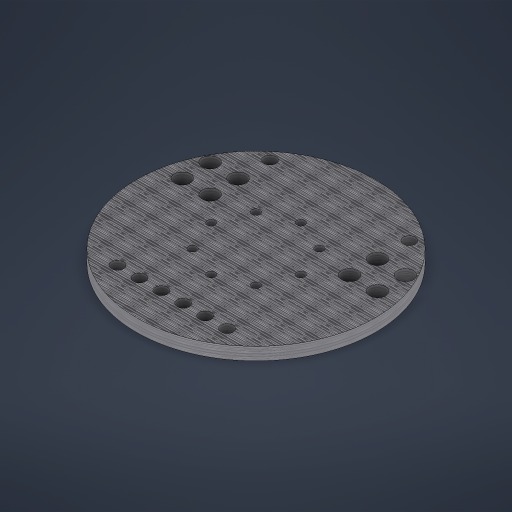
# Autodesk Inventor part: TurretBasePlate
Saved by Autodesk Inventor 2024 (Build 280153000, 153)
## iProperties
Created: 2023-11-22
Part Number: TurretBasePlate
Material: Generic
Document SubType Name: Modeling
Designer: avsar
Density: 1 g/cm^3
Appearance: Machined 03
Author: avsar
Autodesk Inventor part; units mm, degrees
ref_plane "YZ Plane" through (0, 0, 0) normal (1, 0, 0) x (0, 1, 0)
ref_plane "XZ Plane" through (0, 0, 0) normal (0, 1, 0) x (-1, 0, 0)
ref_plane "XY Plane" through (0, 0, 0) normal (0, 0, 1) x (1, 0, 0)
sketch "Sketch1" plane through (0, 0, 0) normal (0, 1, 0) x (-1, 0, 0)
  circle A0 centre (0, 0) radius 60
  dimension "d0" = 120
  constraints: 1 centre point, 1 coincident
  measures "d0" diameter of A0
extrude "Extrusion1" add sketch "Sketch1" along normal mid plane 6.35
sketch "Sketch2" plane through (0, 3.175, 0) normal (0, 1, 0) x (1, 0, 0)
  circle A0 centre (0, 22.5) radius 2
  circle A1 centre (-15.9099, 15.9099) radius 2
  circle A2 centre (-22.5, 0) radius 2
  circle A3 centre (-15.9099, -15.9099) radius 2
  circle A4 centre (0, -22.5) radius 2
  circle A5 centre (15.9099, -15.9099) radius 2
  circle A6 centre (22.5, 0) radius 2
  circle A7 centre (15.9099, 15.9099) radius 2
  point P0 (0, 0)
  dimension "d3" = 4
  dimension "d4" = 22.5
  dimension "d7" = 360
  constraints: 8 centre point, 1 vertical alignment, 17 other
  measures "d3" diameter of A0
  measures "d4" distance of point (0, 0) A0.centre
extrude "Extrusion2" cut sketch "Sketch2" against normal through all
sketch "Sketch3" plane through (0, 3.175, 0) normal (0, 1, 0) x (1, 0, 0)
  circle A0 centre (-42, 20) radius 2.5 construction
  circle A1 centre (-48, 26) radius 2 construction
  circle A2 centre (-48, 14) radius 2 construction
  circle A3 centre (-36, 14) radius 2 construction
  circle A4 centre (-36, 26) radius 2 construction
  circle A5 centre (0, 0) radius 60 construction
  line L0 (0, 60) -> (0, -60) construction
  circle A6 centre (42, 20) radius 2.5 construction
  circle A7 centre (48, 26) radius 2 construction
  circle A8 centre (48, 14) radius 2 construction
  circle A9 centre (36, 14) radius 2 construction
  circle A10 centre (36, 26) radius 2 construction
  circle A11 centre (-20, -42) radius 2.5 construction
  circle A12 centre (-25, -37) radius 2 construction
  circle A13 centre (-25, -47) radius 2 construction
  circle A14 centre (-15, -47) radius 2 construction
  circle A15 centre (-15, -37) radius 2 construction
  circle A16 centre (20, -42) radius 2.5 construction
  circle A17 centre (25, -37) radius 2 construction
  circle A18 centre (25, -47) radius 2 construction
  circle A19 centre (15, -47) radius 2 construction
  circle A20 centre (15, -37) radius 2 construction
  circle A21 centre (-27.5, -42) radius 3
  line L1 (-60, 0) -> (60, 0) construction
  circle A22 centre (-16.5, -42) radius 3
  circle A23 centre (-5.5, -42) radius 3
  circle A24 centre (5.5, -42) radius 3
  circle A25 centre (16.5, -42) radius 3
  circle A26 centre (27.5, -42) radius 3
  line L2 (-5.5, -42) -> (5.5, -42) construction
  point P0 (0, -42)
  dimension "d11" = 5
  dimension "d12" = 42
  dimension "d13" = 20
  dimension "d14" = 4
  dimension "d15" = 6
  dimension "d16" = 6
  dimension "d19" = 360
  dimension "d23" = 5
  dimension "d24" = 42
  dimension "d25" = 20
  dimension "d26" = 4
  dimension "d27" = 5
  dimension "d28" = 5
  dimension "d31" = 360
  dimension "d49" = 6
  dimension "d52" = 11
  constraints: 26 centre point, 10 symmetric about line, 6 end point, 4 point on circle, 3 horizontal, 3 midpoint, 1 coincident, 1 horizontal alignment, 1 vertical, 1 vertical alignment, 38 other
  measures "d11" diameter of A0
  measures "d12" horizontal distance of point (0, 0) A0.centre
  measures "d13" vertical distance of point (0, 0) A0.centre
  measures "d14" diameter of A1
  measures "d15" horizontal distance of A1.centre A0.centre
  measures "d16" horizontal distance of A0.centre A1.centre
  measures "d23" diameter of A11
  measures "d24" vertical distance of point (0, 0) A11.centre
  measures "d25" horizontal distance of point (0, 0) A11.centre
  measures "d26" diameter of A12
  measures "d27" horizontal distance of A11.centre A12.centre
  measures "d28" horizontal distance of A11.centre A12.centre
  measures "d49" diameter of A21
  measures "d52" distance of A21.centre A22.centre
extrude "Extrusion3" cut sketch "Sketch3" against normal through all
sketch "Sketch4" plane through (0, 3.175, 0) normal (0, 1, 0) x (1, 0, 0)
  circle A0 centre (-49, 42) radius 3 construction
  circle A1 centre (-49, 26) radius 4
  circle A2 centre (-49, 12) radius 4
  circle A3 centre (0, 0) radius 60 construction
  line L0 (-60, 0) -> (60, 0) construction
  circle A4 centre (-35, 42) radius 3
  circle A5 centre (-35, 26) radius 4
  circle A6 centre (-35, 12) radius 4
  line L1 (0, 60) -> (0, 0) construction
  circle A7 centre (49, 26) radius 4
  circle A8 centre (49, 12) radius 4
  circle A9 centre (35, 42) radius 3
  circle A10 centre (35, 26) radius 4
  circle A11 centre (35, 12) radius 4
  dimension "d33" = 6
  dimension "d34" = 8
  dimension "d35" = 8
  dimension "d36" = 16
  dimension "d37" = 14
  dimension "d40" = 14
  dimension "d45" = 35
  dimension "d46" = 12
  constraints: 11 centre point, 5 symmetric about line, 4 end point, 3 point on circle, 2 horizontal, 2 vertical alignment, 1 coincident, 1 midpoint, 1 vertical, 11 other
  measures "d33" diameter of A0
  measures "d34" diameter of A1
  measures "d35" diameter of A2
  measures "d36" distance of A0.centre A1.centre
  measures "d37" distance of A2.centre A1.centre
  measures "d40" distance of A0.centre A4.centre
  measures "d45" horizontal distance of point (0, 0) A6.centre
  measures "d46" vertical distance of point (0, 0) A6.centre
extrude "Extrusion4" cut sketch "Sketch4" against normal through all
body "Solid1"
